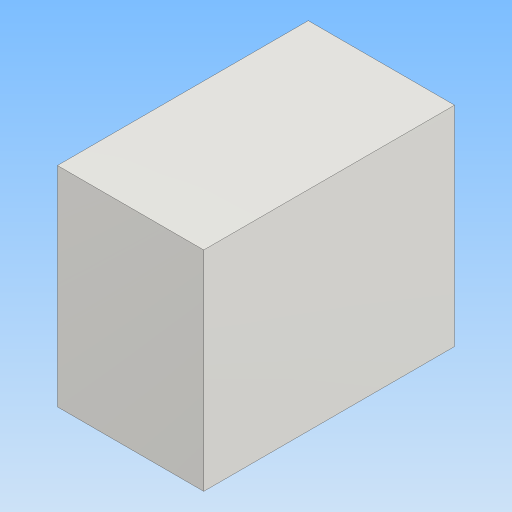
# Autodesk Inventor part: Wellennut_Verbindung_Deck_Antrieb
Saved by Autodesk Inventor 2024.4 (Build 284460000, 460)
## iProperties
Created: 2026-01-22
Part Number: Wellennut_Verbindung_Deck_Antrieb
Material: Generisch
Document SubType Name: Modeling
Designer: windows-desktop
Mass: 0.84 g
Surface Area: 5.48 cm^2
Volume: 0.84 cm^3
Density: 1 g/cm^3
Appearance: Vorgabe
Masse[kg]: 0,0008 kg
Author: windows-desktop
Autodesk Inventor part; units mm, degrees
ref_plane "YZ Plane" through (0, 0, 0) normal (1, 0, 0) x (0, 1, 0)
ref_plane "XZ Plane" through (0, 0, 0) normal (0, 1, 0) x (-1, 0, 0)
ref_plane "XY Plane" through (0, 0, 0) normal (0, 0, 1) x (1, 0, 0)
sketch "Skizze1" plane through (0, 0, 0) normal (0, 1, 0) x (-1, 0, 0)
  line L0 (3.3495, 5.2002) -> (-3.6505, 5.2002)
  line L1 (-3.6505, 5.2002) -> (-3.6505, -4.7998)
  line L2 (-3.6505, -4.7998) -> (3.3495, -4.7998)
  line L3 (3.3495, -4.7998) -> (3.3495, 5.2002)
  point P0 (0, 0)
  dimension "d0" = 7
  dimension "d1" = 10
  constraints: 8 end point, 2 parallel, 1 horizontal, 1 perpendicular
  measures "d0" distance of L2.end L1.end
  measures "d1" distance of L1.end L0.end
extrude "Extrusion1" add sketch "Skizze1" along normal blind 12
